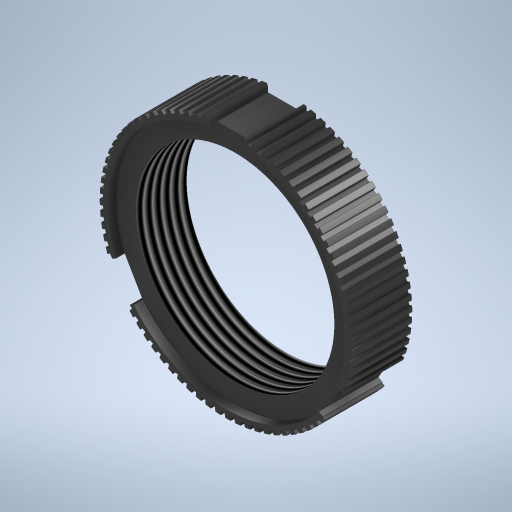
# Autodesk Inventor part: PORCA DO BOTÃO
Saved by Autodesk Inventor 2023 (Build 270158000, 158)
## iProperties
Created: 2023-10-18
Part Number: PORCA DO BOTÃO
Material: Genérico
Document SubType Name: Modeling
Designer: vinicius.sena
Density: 1 g/cm^3
Appearance: Padrão
Author: vinicius.sena
Autodesk Inventor part; units mm, degrees
ref_plane "YZ Plane" through (0, 0, 0) normal (1, 0, 0) x (0, 1, 0)
ref_plane "XZ Plane" through (0, 0, 0) normal (0, 1, 0) x (-1, 0, 0)
ref_plane "XY Plane" through (0, 0, 0) normal (0, 0, 1) x (1, 0, 0)
sketch "Esboço1" plane through (0, 0, 0) normal (0, 0, 1) x (1, 0, 0)
  circle A0 centre (0, 0) radius 14
  dimension "d0" = 28
  constraints: 1 centre point, 1 coincident
  measures "d0" diameter of A0
extrude "Extrusão1" add sketch "Esboço1" along normal blind 6.6
sketch "Esboço2" plane through (0, 0, 6.6) normal (0, 0, 1) x (1, 0, 0)
  circle A0 centre (0, 0) radius 11
  dimension "d3" = 22
  constraints: 1 centre point, 1 coincident
  measures "d3" diameter of A0
extrude "Extrusão2" cut sketch "Esboço2" against normal through all
thread "Rosca1" size "M22x1" class "6H" standard "ANSI Metric M Profile" length 15
sketch "Esboço3" plane through (0, 0, 6.6) normal (0, 0, 1) x (1, 0, 0)
  line L0 (-2, 15) -> (2, 15)
  line L1 (2, 15) -> (2, 13)
  line L2 (2, 13) -> (-2, 13)
  line L3 (-2, 13) -> (-2, 15)
  circle A0 centre (0, 0) radius 14 projected
  line L4 (-2, 15) -> (2, 13) construction
  line L5 (2, 15) -> (-2, 13) construction
  line L6 (12.1262, -6.9969) -> (-12.1226, -7.0031)
  line L7 (-12.1226, -7.0031) -> (-0.0036, 14)
  line L8 (-0.0036, 14) -> (12.1262, -6.9969)
  line L9 (11.9922, -9.2289) -> (10.2601, -8.2289)
  line L10 (10.2601, -8.2289) -> (12.2601, -4.7648)
  line L11 (12.2601, -4.7648) -> (13.9922, -5.7648)
  line L12 (13.9922, -5.7648) -> (11.9922, -9.2289)
  line L13 (11.1262, -4.9969) -> (13.1262, -8.9969) construction
  line L14 (13.1262, -4.9969) -> (11.1262, -8.9969) construction
  line L15 (-13.9886, -5.7711) -> (-12.2565, -4.7711)
  line L16 (-12.2565, -4.7711) -> (-10.2565, -8.2352)
  line L17 (-10.2565, -8.2352) -> (-11.9886, -9.2352)
  line L18 (-11.9886, -9.2352) -> (-13.9886, -5.7711)
  line L19 (-13.1226, -5.0031) -> (-11.1226, -9.0031) construction
  line L20 (-11.1226, -5.0031) -> (-13.1226, -9.0031) construction
  point P0 (0, 14)
  dimension "d8" = 4
  dimension "d9" = 2
  dimension "d12" = 2
  dimension "d13" = 4
  dimension "d14" = 2
  dimension "d15" = 4
  constraints: 42 end point, 6 midpoint, 6 parallel, 3 perpendicular, 2 point on circle, 1 coincident, 1 horizontal, 7 other
  measures "d8" distance of L1.end L2.end
  measures "d9" distance of L0.end L1.end
  measures "d12" distance of L10.end L11.end
  measures "d13" distance of L9.end L10.end
  measures "d14" distance of L16.end L17.end
  measures "d15" distance of L15.end L16.end
extrude "Extrusão3" cut sketch "Esboço3" against normal through all contours L0 L1 A0 L3 | A0 L7 L2 L3 | L1 L2 L8 A0 | L8 L2 L7 | L15 L16 L7 A0 | A0 L17 L18 L15 | L6 L16 L17 A0 | L7 L16 L6 | L11 L12 L9 A0 | A0 L8 L10 L11 | L8 L6 L10 | A0 L9 L10 L6
sketch "Esboço4" plane through (0, 0, 6.6) normal (0, 0, 1) x (1, 0, 0)
  line L0 (-13.6414, -3.8386) -> (-13.2084, -3.5886)
  line L1 (-13.2084, -3.5886) -> (-12.9584, -4.0216)
  line L2 (-12.9584, -4.0216) -> (-13.3914, -4.2716)
  line L3 (-13.3914, -4.2716) -> (-13.6414, -3.8386)
  line L4 (-13.6414, -3.8386) -> (-12.9584, -4.0216) construction
  line L5 (-13.2084, -3.5886) -> (-13.3914, -4.2716) construction
  line L6 (-12.9987, -5.1995) -> (-12.2565, -4.7711) projected
  point P0 (0, 0)
  point P1 (-13.2999, -3.9301)
  point P2 (-12.6276, -4.9853)
  dimension "d18" = 0.5
  dimension "d19" = 0.5
  dimension "d24" = 1
  constraints: 12 end point, 3 midpoint, 2 parallel, 1 perpendicular
  measures "d18" distance of L1.end L2.end
  measures "d19" distance of L0.end L1.end
  measures "d24" distance between parallel lines of L6 L2
extrude "Extrusão4" cut sketch "Esboço4" against normal through all
pattern_circular "Padrão circular1" count 80 over 360 about axis through (0, 0, 0) along (0, 0, 1) of "Extrusão4"
sketch "Esboço5" plane through (0, 0, 6.6) normal (0, 0, 1) x (1, 0, 0)
  circle A0 centre (0, 0) radius 11
  circle A1 centre (0, 0) radius 13.15
  dimension "d30" = 22
  dimension "d31" = 26.3
  constraints: 2 centre point, 2 coincident
  measures "d30" diameter of A0
  measures "d31" diameter of A1
extrude "Extrusão5" cut sketch "Esboço5" against normal blind 1
